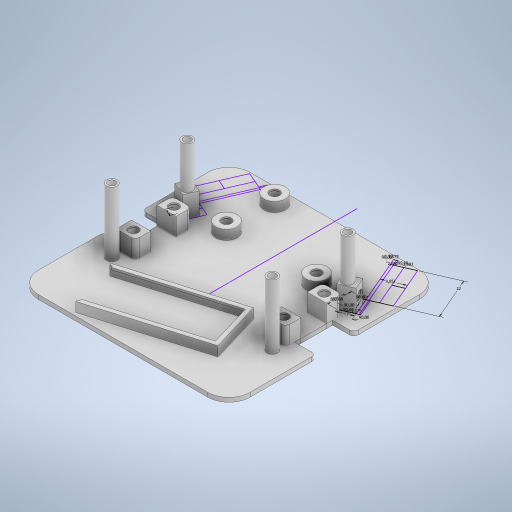
# Autodesk Inventor part: heheheha
Saved by Autodesk Inventor 2023 (Build 270158000, 158)
## iProperties
Created: 2022-12-15
Part Number: heheheha
Material: Ogólny
Document SubType Name: Modeling
Designer: User
Density: 1 g/cm^3
Appearance: Domyślna
Author: User
Autodesk Inventor part; units mm, degrees
ref_plane "YZ Plane" through (0, 0, 0) normal (1, 0, 0) x (0, 1, 0)
ref_plane "XZ Plane" through (0, 0, 0) normal (0, 1, 0) x (-1, 0, 0)
ref_plane "XY Plane" through (0, 0, 0) normal (0, 0, 1) x (1, 0, 0)
sketch "Szkic2" plane through (0, 0, 0) normal (0, 1, 0) x (-1, 0, 0)
  line L0 (50, -50) -> (-50, -50)
  line L1 (50, -50) -> (50, 50)
  line L2 (0, -53.6442) -> (0, 78.3558)
  line L3 (50, 50) -> (-50, 50)
  line L4 (-50, -50) -> (-50, 50)
  line L5 (67.5466, 0) -> (-74.1589, 0)
  line L6 (50, -9) -> (40, -9)
  line L7 (40, -9) -> (40, 9)
  line L8 (40, 9) -> (50, 9)
  line L9 (50, 9) -> (50, -9)
  line L10 (-50, -9) -> (-40, -9)
  line L11 (-40, -9) -> (-40, 9)
  line L12 (-40, 9) -> (-50, 9)
  line L13 (-50, 9) -> (-50, -9)
  line L14 (40, -7.5) -> (31, -7.5)
  line L15 (31, -7.5) -> (31, 7.5)
  line L16 (31, 7.5) -> (40, 7.5)
  line L17 (40, 7.5) -> (40, -7.5)
  line L18 (-40, -7.5) -> (-28.5, -7.5)
  line L19 (-28.5, -7.5) -> (-28.5, 7.5)
  line L20 (-28.5, 7.5) -> (-40, 7.5)
  line L21 (-40, 7.5) -> (-40, -7.5)
  line L22 (31.5, 9) -> (-31.5, 9)
  line L23 (31, 7.5) -> (31, 9)
  line L24 (-28.5, 7.5) -> (-28.5, 9)
  line L25 (31.5, -9) -> (-31.5, -9)
  line L26 (-28.5, -7.5) -> (-28.5, -9)
  line L27 (31, -7.5) -> (31, -9)
  line L28 (40, -11.25) -> (40, -9)
  line L29 (40, 11.25) -> (40, 9)
  line L30 (-40, -11.25) -> (-40, -9)
  line L31 (-40, 11.25) -> (-40, 9)
  line L32 (40, -9) -> (40, -7.5)
  line L33 (-40, -9) -> (-40, -7.5)
  line L34 (40, 9) -> (40, 7.5)
  line L35 (-40, 9) -> (-40, 7.5)
  line L36 (40, -9) -> (40, -9)
  line L37 (40, 9) -> (40, 9)
  line L38 (-40, -9) -> (-40, -9)
  line L39 (-40, 9) -> (-40, 9)
  line L40 (40, -14.25) -> (40, -13.75)
  line L41 (31, 5.5681) -> (31, 11.25)
  line L42 (33, 13.25) -> (38, 13.25)
  line L43 (40, 14.25) -> (40, 13.75)
  line L44 (-40, -14.25) -> (-40, -13.75)
  line L45 (-31, 9) -> (-31, 11.25)
  line L46 (-40, 14.25) -> (-40, 14.75)
  line L47 (50, -50) -> (50, 50)
  line L48 (50, -50) -> (-50, -50)
  line L49 (50, -9) -> (40, -9)
  line L50 (40, 9) -> (50, 9)
  line L51 (40, 7.5) -> (40, -7.5)
  line L52 (50, -50) -> (-50, -50)
  line L53 (-40, 0) -> (-9.8, 0)
  line L54 (-9.7869, 9) -> (-9.7869, -9)
  line L55 (9.7869, 9) -> (9.7869, -9)
  line L56 (40, -6) -> (31, -6)
  line L57 (40, 6) -> (31, 6)
  line L58 (40, -13.75) -> (40, -9)
  line L59 (31, -5.5681) -> (31, -11.25)
  line L60 (33, -13.25) -> (38, -13.25)
  line L61 (-40, -7.5) -> (-31, -7.5)
  line L62 (-31, 7.5) -> (-40, 7.5)
  line L63 (-31, 5.5681) -> (-31, 13.25)
  line L64 (-33, 13.25) -> (-38, 13.25)
  line L65 (-40, -6) -> (-31, -6)
  line L66 (-33, -13.25) -> (-38, -13.25)
  line L67 (-31, -5.5681) -> (-31, -11.25)
  arc A0 (38, -13.25) -> (40, -11.25) centre (38, -11.25) ccw
  arc A1 (31, -11.25) -> (33, -13.25) centre (33, -11.25) ccw
  arc A2 (40, 11.25) -> (38, 13.25) centre (38, 11.25) ccw
  arc A3 (33, 13.25) -> (31, 11.25) centre (33, 11.25) ccw
  arc A4 (-31, 11.25) -> (-33, 13.25) centre (-33, 11.25) ccw
  arc A5 (-38, 13.25) -> (-40, 11.25) centre (-38, 11.25) ccw
  arc A6 (-40, -11.25) -> (-38, -13.25) centre (-38, -11.25) ccw
  arc A7 (-33, -13.25) -> (-31, -11.25) centre (-33, -11.25) ccw
  line L68 (-40, 6) -> (-31, 6)
  circle A8 centre (35.5, 10.125) radius 1.6547
  circle A9 centre (35.5, -10.125) radius 1.6547
  circle A10 centre (-35.5, 10.125) radius 1.6547
  circle A11 centre (-35.5, -10.125) radius 1.6547
  point P0 (0, 0)
  point P1 (-50, 9)
  point P2 (-34.25, -7.5)
  point P3 (31.5, -9)
  point P4 (31.5, -9)
  point P5 (-31.5, 9)
  point P6 (-31.5, 9)
  point P7 (40, 7.5)
  point P8 (31, 13.25)
  point P9 (40.0775, 13.25)
  point P10 (-31, -9)
  point P11 (-31, -14.25)
  point P12 (-31, 15.2922)
  point P13 (-31, 9)
  point P14 (31, 9)
  point P15 (-50, 0)
  point P16 (31, -13.25)
  point P17 (40.0775, -13.25)
  point P18 (-40.0775, 13.25)
  point P19 (-31, -13.25)
  point P20 (-40.0775, -13.25)
  dimension "d30" = 100
  dimension "d31" = 132
  dimension "d32" = 18
  dimension "d33" = 10
  dimension "d38" = 9
  dimension "d39" = 15
  dimension "d40" = 15
  dimension "d41" = 11.5
  dimension "d42" = 10
  dimension "d44" = 15
  dimension "d47" = 0
  dimension "d62" = 0.5
  dimension "d68" = 100
  dimension "d69" = 50
  dimension "d70" = 30.2
  dimension "d71" = 1.5
  dimension "d73" = 5.75
  dimension "d74" = 2
  constraints: 134 end point, 35 symmetric about line, 28 point on line, 16 point on circle, 16 tangent, 14 horizontal, 12 centre point, 12 vertical, 9 parallel, 7 equal radius, 7 midpoint, 6 perpendicular, 1 collinear, 64 other
  measures "d30" distance of L0.start L0.end
  measures "d31" distance of L2.start L2.end
  measures "d32" distance of L6.end L7.end
  measures "d33" distance of L6.start L6.end
  measures "d38" distance of L14.start L14.end
  measures "d39" distance of L14.end L15.end
  measures "d40" distance of L20.end L18.start
  measures "d41" distance of L18.start L18.end
  measures "d42" distance of L10.start L10.end
  measures "d44" distance from line of L20 point (-34.25, -7.5)
  measures "d47" distance of L6.end L32.start
  measures "d62" distance of L44.end L44.start
  measures "d68" distance of L0.end L3.end
  measures "d69" distance of point (-50, 0) L3.end
  measures "d70" distance of L53.start L53.end
  measures "d71" distance between parallel lines of L56 L14
  measures "d73" distance between parallel lines of L60 L14
  measures "d74" radius of A0
extrude "Wyciągnięcie proste3" add sketch "Szkic2" along normal blind 10.5 contours L28 A0 L60 A1 L59 L27 L14 L7 | L14 L15 L56 L7 | L11 L18 L67 A7 L66 A6 L30 | L7 L16 L23 L41 A3 L42 A2 L29 | L57 L15 L16 L7 | L11 L65 L67 L18 | L31 A5 L64 A4 L45 L63 L20 L11 | L11 L20 L63 L68 | A8 | A9 | A10 | A11
extrude "Wyciągnięcie proste4" add sketch "Szkic2" along normal blind 2 separate body contours L0 L2 L25 L59 A1 L60 A0 L28 L6 L1 | L0 L4 L10 L30 A6 L66 A7 L67 L25 L2 | L25 L54 L5 L2 | L2 L5 L55 L25 | L28 A0 L60 A1 L59 L27 L14 L7 | L5 L54 L22 L2 | L2 L22 L55 L5 | L55 L5 L15 L27 L25 | L25 L26 L19 L5 L54 | L8 L29 A2 L42 A3 L41 L22 L2 L3 L1 | L7 L56 L15 L5 | L5 L15 L57 L7 | L14 L15 L56 L7 | L11 L18 L67 A7 L66 A6 L30 | L22 L45 A4 L64 A5 L31 L12 L4 L3 L2 | L55 L22 L23 L15 L5 | L5 L19 L24 L22 L54 | L25 L67 L18 L26 | L7 L16 L23 L41 A3 L42 A2 L29 | L57 L15 L16 L7 | L11 L68 L63 L20 L19 L5 | L5 L19 L18 L67 L65 L11 | L11 L65 L67 L18 | L31 A5 L64 A4 L45 L63 L20 L11 | L11 L20 L63 L68 | L24 L20 L63 L22 | A8 | A9 | A10 | A11
fillet "Zaokrąglenie4" radius 10 4 edges at (-50, 1, -50) (-50, 1, 50) (50, 1, 50) (50, 1, -50)
fillet "Zaokrąglenie5" radius 2 4 edges at (50, 1, 9) (50, 1, -9) (-50, 1, 9) (-50, 1, -9)
sketch "Szkic5" plane through (0, 2, 0) normal (0, 1, 0) x (1, 0, 0)
  line L0 (24.5, 7.6836) -> (-24.5, 7.6836)
  line L1 (-24.5, 7.6836) -> (-24.5, 47.6836)
  line L2 (-24.5, 47.6836) -> (24.5, 47.6836)
  line L3 (24.5, 47.6836) -> (24.5, 7.6836)
  line L4 (0, -42.3954) -> (0, 57.9871)
  line L5 (67.9051, 0) -> (-103.5521, 0)
  circle A0 centre (-21.3, 42.9106) radius 5
  circle A1 centre (-21.3, 20.1106) radius 5
  circle A2 centre (21.3, 20.1106) radius 5
  line L6 (26.631, -32.4148) -> (-23.1992, -47.2793)
  line L7 (-23.1992, -47.2793) -> (-29.7739, -25.239)
  line L8 (-29.7739, -25.239) -> (20.0563, -10.3745)
  line L9 (20.0563, -10.3745) -> (26.631, -32.4148)
  line L10 (27.8751, -33.0872) -> (-23.8716, -48.5234)
  line L11 (-23.8716, -48.5234) -> (-31.018, -24.5666)
  line L12 (-31.018, -24.5666) -> (20.7287, -9.1304)
  line L13 (20.7287, -9.1304) -> (27.8751, -33.0872)
  line L14 (-23.1992, -47.2793) -> (-24.1575, -47.5652)
  line L15 (-29.7739, -25.239) -> (-30.7321, -25.5249)
  line L16 (26, -27.2838) -> (-27, -27.2838)
  circle A3 centre (-21.3, 42.9106) radius 1.75
  line L17 (-4.8588, -17.8068) -> (1.7159, -39.8471)
  point P0 (0, 0)
  point P1 (0, 7.7958)
  point P2 (0, -16.3574)
  point P3 (0, -15.3139)
  point P4 (0, -41.4025)
  point P5 (0, -40.3589)
  point P6 (0, -27.2838)
  point P7 (3.6487, -26.2263)
  dimension "d75" = 40
  dimension "d76" = 49
  dimension "d78" = 10
  dimension "d79" = 10
  dimension "d86" = 52
  dimension "d87" = 23
  dimension "d88" = 26.631
  dimension "d89" = 1
  dimension "d90" = 1
  dimension "d91" = 1
  dimension "d92" = 1
  dimension "d114" = 3.5
  dimension "d115" = 22.8
  dimension "d123" = 24.5
  dimension "d124" = 42.6
  constraints: 36 end point, 6 parallel, 5 perpendicular, 4 centre point, 4 point on line, 3 horizontal, 3 midpoint, 2 vertical, 1 coincident, 1 symmetric about line
  measures "d75" distance of L2.end L0.start
  measures "d76" distance of L0.start L0.end
  measures "d78" diameter of A0
  measures "d79" diameter of A1
  measures "d86" distance of L7.end L8.end
  measures "d87" distance of L6.end L7.end
  measures "d88" distance from line of L4 L6.start
  measures "d89" distance between parallel lines of L6 L10
  measures "d90" distance between parallel lines of L9 L13
  measures "d91" distance between parallel lines of L7 L11
  measures "d92" distance between parallel lines of L8 L12
  measures "d114" diameter of A3
  measures "d115" distance of A1.centre A0.centre
  measures "d123" distance from line of L4 L0.end
  measures "d124" distance of A2.centre A1.centre
extrude "Wyciągnięcie proste5" add sketch "Szkic5" along normal blind 3.5 contours L10 L11 L14 L6 L4 | L4 L6 L9 L8 L12 L13 L10 | L15 L11 L12 L4 L8 bodies 2
sketch "Szkic7" plane through (0, 5.5, 0) normal (0, 1, 0) x (1, 0, 0)
  line L0 (-31.018, -24.5666) -> (20.7287, -9.1304) projected
  line L1 (-23.8716, -48.5234) -> (-24.1575, -47.5652) projected
  line L2 (20.0563, -10.3745) -> (26.631, -32.4148) projected
  line L3 (26.631, -32.4148) -> (-24.1575, -47.5652) projected
  line L4 (-30.7321, -25.5249) -> (20.0563, -10.3745) projected
  line L5 (27.8751, -33.0872) -> (-23.8716, -48.5234) projected
  line L6 (20.7287, -9.1304) -> (27.8751, -33.0872)
  line L7 (27.8751, -33.0872) -> (-23.8716, -48.5234)
  line L8 (-23.8716, -48.5234) -> (-31.018, -24.5666)
  line L9 (-31.018, -24.5666) -> (20.7287, -9.1304)
  line L10 (20.0563, -10.3745) -> (-30.7321, -25.5249) projected
  line L11 (26.631, -32.4148) -> (20.0563, -10.3745) projected
  line L12 (20.0563, -10.3745) -> (26.631, -32.4148)
  line L13 (26.631, -32.4148) -> (-23.1992, -47.2793)
  line L14 (-23.1992, -47.2793) -> (-29.7739, -25.239)
  line L15 (-29.7739, -25.239) -> (20.0563, -10.3745)
  line L16 (19.098, -10.6604) -> (25.6727, -32.7007)
  line L17 (19.3839, -11.6187) -> (-29.488, -26.1973)
  line L18 (25.3869, -31.7424) -> (-23.485, -46.321)
  point P0 (0, 0)
  point P1 (22.3854, -21.6805)
  point P2 (-31.018, -24.5666)
  point P3 (-29.7739, -25.239)
  point P4 (-23.1992, -47.2793)
  dimension "d177" = 1
  dimension "d178" = 1
  dimension "d179" = 1
  constraints: 22 end point, 6 perpendicular, 6 point on line, 5 equal length, 1 midpoint
  measures "d177" distance from line of point (22.385, -21.681) L2
  measures "d178" distance between parallel lines of L17 L15
  measures "d179" distance between parallel lines of L13 L18
extrude "Wyciągnięcie proste7" add sketch "Szkic7" along normal blind 1 contours L0 L6 L5 L1 L3 L2 L4 L8 | L4 L16 L17 L14 | L4 L2 L3 L16 | L14 L18 L16 L3 bodies 2
extrude "Wyciągnięcie proste8" add sketch "Szkic5" along normal blind 4.5 contours A2 L3 | L3 A2 | A1 L1 | L1 A1 | A0 L1 L2 | L2 A0 | A0 L1 | A3 picked at (-24.0167, 42.9106) bodies 2
sketch "Szkic8" plane through (-21.3, 6.5, -42.9106) normal (0, 1, 0) x (1, 0, 0)
  circle A0 centre (0, -22.8) radius 5 projected
  circle A1 centre (0, 0) radius 5 projected
  circle A2 centre (42.6, -22.8) radius 5 projected
  point P0 (21.3, -42.9106)
  point P1 (0, -22.8)
  constraints: 3 coincident
hole "Otwór2" at (21.3, 6.5, -20.1106) at (-21.3, 6.5, -42.9106) at (-21.3, 6.5, -20.1106) direction (0, -1, 0) diameter 4 depth 4 counterbore diameter 4.5 counterbore depth 0.6 bodies 2
sketch "Szkic10" plane through (0, 2, 0) normal (0, 1, 0) x (1, 0, 0)
  line L0 (30.6682, 45.4835) -> (39.7138, 49.3848)
  line L1 (39.7138, 49.3848) -> (48.4264, 29.1835)
  line L2 (48.4264, 29.1835) -> (39.3808, 25.2823)
  line L3 (39.3808, 25.2823) -> (30.6682, 45.4835)
  line L4 (32.1145, 46.1073) -> (30.9335, 48.8455)
  line L5 (30.9335, 48.8455) -> (29.4873, 48.2217)
  line L6 (29.4873, 48.2217) -> (30.6682, 45.4835)
  line L7 (35.191, 47.4342) -> (43.9036, 27.2329)
  line L8 (39.5473, 37.3335) -> (44.0701, 39.2842)
  line L9 (44.2937, 17.868) -> (42.8475, 17.2443)
  line L10 (39.3808, 25.2823) -> (42.8475, 17.2443)
  line L11 (44.2937, 17.868) -> (40.827, 25.906)
  line L12 (30.4882, 48.6534) -> (31.6691, 45.9152)
  line L13 (31.6691, 45.9152) -> (43.8484, 17.676)
  line L14 (0, 60.4183) -> (0, -9.1824)
  line L15 (-30.6683, 45.4835) -> (-39.7138, 49.3848)
  line L16 (-39.7138, 49.3848) -> (-48.4264, 29.1835)
  line L17 (-48.4264, 29.1835) -> (-39.3808, 25.2823)
  line L18 (-39.3808, 25.2823) -> (-30.6683, 45.4835)
  line L19 (-32.1145, 46.1073) -> (-30.9335, 48.8455)
  line L20 (-30.9335, 48.8455) -> (-29.4873, 48.2217)
  line L21 (-29.4873, 48.2217) -> (-30.6683, 45.4835)
  line L22 (-35.191, 47.4342) -> (-43.9036, 27.2329)
  line L23 (-39.5473, 37.3335) -> (-44.0701, 39.2842)
  line L24 (-39.3808, 25.2823) -> (-42.8475, 17.2443)
  line L25 (-44.2938, 17.868) -> (-40.8271, 25.906)
  line L26 (-30.4882, 48.6534) -> (-31.6691, 45.9152)
  line L27 (-31.6691, 45.9152) -> (-43.8484, 17.676)
  line L28 (-44.2938, 17.868) -> (-42.8475, 17.2443)
  line L29 (42.8475, 17.2443) -> (36.4198, 14.4721)
  line L30 (38, 13.25) -> (33, 13.25) projected
  line L31 (36.4198, 14.4721) -> (32.9531, 22.5101)
  line L32 (39.3808, 25.2823) -> (32.9531, 22.5101)
  line L33 (-42.8475, 17.2443) -> (-36.4199, 14.4721)
  line L34 (-36.4199, 14.4721) -> (-32.9532, 22.5101)
  line L35 (-39.3808, 25.2823) -> (-32.9532, 22.5101)
  line L36 (-40.1755, 16.0918) -> (-36.7088, 24.1298)
  circle A0 centre (-38.4421, 20.1108) radius 2
  line L37 (34.0437, 19.9815) -> (40.4714, 22.7537)
  line L38 (-34.0437, 19.9815) -> (-40.4714, 22.7537)
  point P0 (0, 0)
  point P1 (-40.3817, 25.714)
  point P2 (40.3817, 25.714)
  point P3 (-34.0437, 19.9815)
  dimension "d134" = 9.851
  dimension "d135" = 22
  dimension "d136" = 2.982
  dimension "d138" = 1.575
  dimension "d140" = 90
  dimension "d141" = 90
  dimension "d142" = 2.982
  dimension "d145" = 1.575
  dimension "d146" = 90
  dimension "d147" = 90
  dimension "d148" = 8.038
  dimension "d149" = 1.09
  dimension "d150" = 90
  dimension "d152" = 8.038
  dimension "d153" = 90
  dimension "d155" = 7
  dimension "d159" = 4
  dimension "d171" = 6
  constraints: 76 end point, 22 symmetric about line, 13 point on line, 7 perpendicular, 5 midpoint, 3 parallel, 1 centre point, 1 vertical, 1 other
  measures "d134" distance between parallel lines of L1 L3
  measures "d135" distance of L0.end L1.end
  measures "d136" distance of L4.start L4.end
  measures "d138" distance of L4.end L5.end
  measures "d140" angle of L0 L4
  measures "d141" angle of L6 L5
  measures "d142" distance from line of L0 L4.end
  measures "d145" distance of L9.start L9.end
  measures "d146" angle of L10 L2
  measures "d147" angle of L9 L10
  measures "d148" vertical distance of L2.end L9.end
  measures "d149" distance from line of L12 L5.end
  measures "d150" angle of L29 L10
  measures "d152" vertical distance of L31.start L31.end
  measures "d153" angle of L29 L31
  measures "d155" distance of L9.end L29.end
  measures "d159" distance from line of L27 L36.start
  measures "d171" distance from line of L37 L9.end
extrude "Wyciągnięcie proste9" add sketch "Szkic10" along normal blind 10.414 contours L10 L29 L31 L37 | L38 A0 L36 L33 L24 | L38 L36 A0 | L36 A0 L38 L34 L33 | L36 L38 A0 picked at (-38.8879, 19.4592) picked at (-38.5981, 19.3373) bodies 2
sketch "Szkic11" plane through (0, 12.414, 0) normal (0, 1, 0) x (1, 0, 0)
  circle A0 centre (-37.932, 18.2314) radius 2.5
  circle A1 centre (-37.932, -17.4185) radius 2.5
  line L0 (0, -60.0206) -> (0, 63.8525)
  circle A2 centre (37.932, 18.2314) radius 2.5
  circle A3 centre (-37.932, -17.4185) radius 1.75
  circle A4 centre (-37.932, 18.2314) radius 1.75
  circle A5 centre (37.932, 18.2314) radius 1.75
  circle A6 centre (37.932, 18.2314) radius 2.5
  circle A7 centre (37.932, -17.4185) radius 2.5
  circle A8 centre (37.932, -17.4185) radius 1.75
  point P0 (0, 0)
  dimension "d163" = 5
  dimension "d170" = 3.5
  dimension "d175" = 75.864
  dimension "d188" = 3.5
  dimension "d189" = 3.5
  constraints: 9 centre point, 2 coincident, 2 end point, 2 symmetric about line, 2 vertical, 2 other
  measures "d163" diameter of A0
  measures "d170" diameter of A3
  measures "d175" distance of A2.centre A0.centre
  measures "d188" diameter of A4
  measures "d189" diameter of A5
extrude "Wyciągnięcie proste11" add sketch "Szkic11" along normal blind 20 contours A0 | A2 bodies 2
extrude "Wyciągnięcie proste12" add sketch "Szkic11" along normal blind 20 and the other way blind 10.5 contours A1 bodies 2
extrude "Wyciągnięcie proste13" add sketch "Szkic11" along normal blind 20 and the other way blind 10.5 contours A7 bodies 2
sketch "Szkic12" plane through (40.4714, 2, -22.7537) normal (0.9182391, 0, -0.3960263) x (-0.3960263, 0, -0.9182391)
  circle A0 centre (-2.75, 5.207) radius 1.75
  line L0 (0, 0) -> (-6, 0) projected
  point P0 (-4.8656, -2)
  dimension "d180" = 5.207
  dimension "d181" = 3.5
  constraints: 1 centre point
  measures "d180" distance from line of L0 A0.centre
  measures "d181" diameter of A0
sketch "Szkic13" plane through (-42.8475, 2, -17.2443) normal (-0.9182391, 0, -0.3960263) x (-0.3960263, 0, 0.9182391)
  circle A0 centre (-2.75, 5.207) radius 1.75
  line L0 (0, 0) -> (-6, 0) projected
  point P0 (-1.1344, -2)
  dimension "d182" = 5.207
  dimension "d183" = 3.5
  constraints: 1 centre point
  measures "d182" distance from line of L0 A0.centre
  measures "d183" diameter of A0
extrude "Wyciągnięcie proste16" add sketch "Szkic11" against normal blind 10.5 contours A8 bodies 2
sketch "Szkic14" plane through (0, 10.5, 0) normal (0, 1, 0) x (1, 0, 0)
  circle A0 centre (35.532, -9.543) radius 2.1428
  line L0 (-58.3928, 0) -> (97.4777, 0)
  line L1 (0, -65.83) -> (0, 98.7532)
  circle A1 centre (35.532, 9.543) radius 2.1428
  circle A2 centre (-35.532, -9.543) radius 2.1428
  circle A3 centre (-35.532, 9.543) radius 2.1428
  point P0 (0, 0)
  constraints: 4 centre point, 4 end point, 3 symmetric about line, 1 horizontal, 1 vertical, 3 other
hole "Otwór3" at (35.532, 10.5, 9.543) at (35.532, 10.5, -9.543) at (-35.532, 10.5, 9.543) at (-35.532, 10.5, -9.543) direction (0, -1, 0) diameter 4 depth 4 counterbore diameter 4.5 counterbore depth 0.6 bodies 1
hole "Otwór4" at (41.5604, 7.207, -20.2286) direction (-0.9182391, 0, 0.3960263) diameter 4 depth 4 counterbore diameter 4.5 counterbore depth 0.6 bodies 2
hole "Otwór5" at (-41.7585, 7.207, -19.7694) direction (0.9182391, 0, 0.3960263) diameter 4 depth 4 counterbore diameter 4.5 counterbore depth 0.6 bodies 2
sketch "Szkic15" plane through (0, 0, 0) normal (0, -1, 0) x (1, 0, 0)
  circle A0 centre (0, 42.2321) radius 4.7292
  line L0 (-60.2085, 0) -> (61.0078, 0)
  circle A1 centre (0, -42.2321) radius 4.7292
  line L1 (0, 56.8682) -> (0, -60.1174)
  point P0 (0, 0)
  constraints: 4 end point, 2 centre point, 1 horizontal, 1 point on line, 1 symmetric about line, 1 vertical, 1 other
extrude "Wyciągnięcie proste17" add sketch "Szkic15" along normal blind 4.5 bodies 2
fillet "Zaokrąglenie7" radius 3.75 2 edges at (-4.7292, -4.5, -42.2321) (-4.7292, -4.5, 42.2321)
